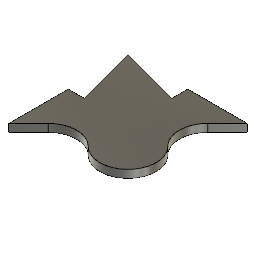
ringing_vfa_01 (Autodesk Fusion 360 design; units mm, degrees)
Autodesk Fusion 360 part; units mm, degrees
sketch "Sketch1" plane through (0, 0, 0) normal (0, 0, 1) x (1, 0, 0) in component "ringing_vfa_01"
  line L0 (0, 0) -> (0, 180) construction
  line L1 (0, 180) -> (-180, 180)
  line L2 (-180, 180) -> (-180, 0)
  line L3 (-180, 0) -> (0, 0) construction
  line L4 (-180, 0) -> (-150, 30)
  arc A0 (-90, 30) -> (-150, 30) centre (-120, 0) ccw
  arc A1 (-90, 30) -> (-30, 90) centre (-60, 60) ccw
  arc A2 (-30, 150) -> (-30, 90) centre (0, 120) ccw
  line L5 (-30, 150) -> (0, 180)
  line L6 (0, 0) -> (-180, 180) construction
  line L7 (-180, 180) -> (-90, 155.8846)
  line L8 (-90, 155.8846) -> (-90, 180)
  line L9 (-180, 180) -> (-155.8846, 90)
  line L10 (-155.8846, 90) -> (-180, 90)
  dimension "d2" = 180
  dimension "d3" = 45
  dimension "d4" = 45
  dimension "d8" = 60
  dimension "d10" = 60
  constraint coincident L0.start L3.end
  constraint tangent L4 A0
  constraint tangent A0 A1
  constraint tangent A1 A2
  constraint tangent A2 L5
  constraint coincident A1.centre L6
  constraint equal A0 A1
  constraint equal A1 A2
  constraint equal L1 L2
  constraint perpendicular L1 L2
  constraint perpendicular L2 L3
  constraint perpendicular L0 L3
  constraint horizontal L3
  constraint coincident L3 A0.centre
  constraint coincident L1 L8.end
  constraint perpendicular L1 L8
  constraint coincident L2 L10.end
  constraint perpendicular L2 L10
  constraint symmetric L6 L7 L9
  constraint midpoint L1 L8.end
  constraint midpoint L2 L10.end
  measures "d2" distance of L0.start L2.end
  measures "d3" angle of L3 L4
  measures "d4" angle of L0 L5
  measures "d8" distance of L2 A0.centre
  measures "d10" angle of L7 L9
extrude "Extrude1" add sketch "Sketch1" along normal blind 12 contours L1 L2 L4 A0 A1 A2 L5 L7 L8 L9 L10 in component "ringing_vfa_01"
component "ringing_vfa_01" placed x (1, 0, 0) y (0, 1, 0) z (0, 0, 1) at (0, 0, 0)
equation "d8 = d2 / 3"
